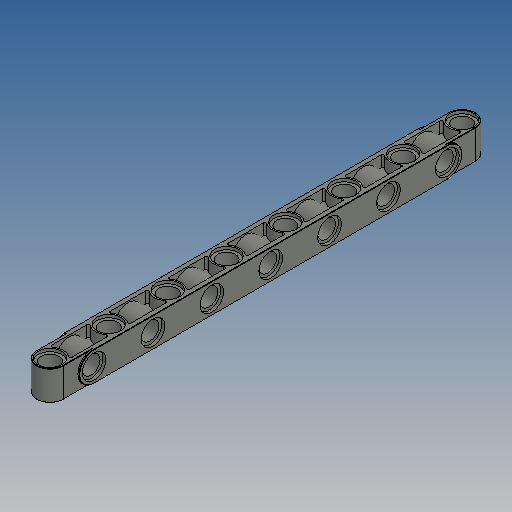
# Autodesk Inventor part: 6330585-Black
Saved by Autodesk Inventor 2025 (Build 290162010, 162A)
## iProperties
Created: 2012-03-21
Part Number: 6330585-Black
Document SubType Name: Modeling
Designer: h.muther
Density: 1.06 g/cm^3
Material: ABS Plastic
Mass: 2.72969 g
Surface Area: 46.8865 cm^2
Volume: 2.57518 cm^3
Appearance: DkBluishGray
Description: Technic, Liftarm 11
Author: h.muther
Autodesk Inventor part; units mm, degrees
ref_plane "YZ Plane" through (0, 0, 0) normal (1, 0, 0) x (0, 1, 0)
ref_plane "XZ Plane" through (0, 0, 0) normal (0, 1, 0) x (-1, 0, 0)
ref_plane "XY Plane" through (0, 0, 0) normal (0, 0, 1) x (1, 0, 0)
sketch "Sketch1" plane through (0, 0, 0) normal (0, 0, 1) x (1, 0, 0)
  line L0 (3.6, -56) -> (3.6, 56)
  line L1 (-3.6, 56) -> (-3.6, -56)
  arc A0 (3.6, 56) -> (-3.6, 56) centre (0, 56) ccw
  arc A1 (-3.6, -56) -> (3.6, -56) centre (0, -56) ccw
  circle A2 centre (0, 56) radius 3.2
  circle A3 centre (0, 56) radius 2.4
  line L2 (2.8, 53.7373) -> (2.8, 42.2627)
  line L3 (-2.8, 53.7373) -> (-2.8, 42.2627)
  arc A4 (-2.8, 53.7373) -> (2.8, 53.7373) centre (0, 56) ccw
  arc A5 (2.8, 42.2627) -> (-2.8, 42.2627) centre (0, 40) ccw
  circle A6 centre (0, 40) radius 3.2
  circle A7 centre (0, 40) radius 2.4
  line L4 (2.8, 37.7373) -> (2.8, 26.2627)
  line L5 (-2.8, 37.7373) -> (-2.8, 26.2627)
  arc A8 (-2.8, 37.7373) -> (2.8, 37.7373) centre (0, 40) ccw
  arc A9 (2.8, 26.2627) -> (-2.8, 26.2627) centre (0, 24) ccw
  circle A10 centre (0, 24) radius 3.2
  circle A11 centre (0, 24) radius 2.4
  line L6 (2.8, 21.7373) -> (2.8, 10.2627)
  line L7 (-2.8, 21.7373) -> (-2.8, 10.2627)
  arc A12 (-2.8, 21.7373) -> (2.8, 21.7373) centre (0, 24) ccw
  arc A13 (2.8, 10.2627) -> (-2.8, 10.2627) centre (0, 8) ccw
  circle A14 centre (0, 8) radius 3.2
  circle A15 centre (0, 8) radius 2.4
  line L8 (2.8, 5.7373) -> (2.8, -5.7373)
  line L9 (-2.8, 5.7373) -> (-2.8, -5.7373)
  arc A16 (-2.8, 5.7373) -> (2.8, 5.7373) centre (0, 8) ccw
  arc A17 (2.8, -5.7373) -> (-2.8, -5.7373) centre (0, -8) ccw
  circle A18 centre (0, -8) radius 3.2
  circle A19 centre (0, -8) radius 2.4
  line L10 (2.8, -10.2627) -> (2.8, -21.7373)
  line L11 (-2.8, -10.2627) -> (-2.8, -21.7373)
  arc A20 (-2.8, -10.2627) -> (2.8, -10.2627) centre (0, -8) ccw
  arc A21 (2.8, -21.7373) -> (-2.8, -21.7373) centre (0, -24) ccw
  circle A22 centre (0, -24) radius 3.2
  circle A23 centre (0, -24) radius 2.4
  circle A24 centre (0, -40) radius 2.4
  circle A25 centre (0, -40) radius 3.2
  line L12 (2.8, -26.2627) -> (2.8, -37.7373)
  arc A26 (2.8, -37.7373) -> (-2.8, -37.7373) centre (0, -40) ccw
  arc A27 (-2.8, -26.2627) -> (2.8, -26.2627) centre (0, -24) ccw
  line L13 (-2.8, -26.2627) -> (-2.8, -37.7373)
  circle A28 centre (0, -56) radius 2.4
  circle A29 centre (0, -56) radius 3.2
  line L14 (2.8, -42.2627) -> (2.8, -53.7373)
  arc A30 (2.8, -53.7373) -> (-2.8, -53.7373) centre (0, -56) ccw
  arc A31 (-2.8, -42.2627) -> (2.8, -42.2627) centre (0, -40) ccw
  line L15 (-2.8, -42.2627) -> (-2.8, -53.7373)
  point P0 (0, 0)
  point P1 (-3.6, 0)
  dimension "d32" = 7.2
  dimension "d48" = 112
  dimension "d49" = 6.4
  dimension "d50" = 4.8
  dimension "d51" = 16
  dimension "d52" = 0.8
  dimension "d55" = 16
  constraints: 32 centre point, 32 end point, 32 point on circle, 17 coincident, 4 equal radius, 4 tangent, 3 horizontal alignment, 3 vertical, 2 vertical alignment, 1 midpoint, 1 parallel, 84 other
  measures "d32" diameter of A0
  measures "d48" distance of A1.centre A0.centre
  measures "d49" diameter of A2
  measures "d50" diameter of A3
  measures "d51" distance of A0.centre A5.centre
  measures "d52" distance between parallel lines of L1 L3
  measures "d55" distance of A7.centre A11.centre
extrude "Extrusion1" add sketch "Sketch1" along normal mid plane 8 contours A1 L1 A0 L0 | A2 | L2 A5 L3 A4 | A6 | L4 A9 L5 A8 | A10 | L6 A13 L7 A12 | A14 | L8 A17 L9 A16 | A18 | L10 A21 L11 A20 | A22 | A25 | L12 A26 L13 A27 | A29 | L14 A30 L15 A31
sketch "Sketch6" plane through (0, 0, 4) normal (0, 0, 1) x (1, 0, 0)
  line L0 (2.8, -10.2627) -> (2.8, -21.7373) projected
  arc A0 (-2.8, -10.2627) -> (2.8, -10.2627) centre (0, -8) ccw projected
  line L1 (-2.8, -10.2627) -> (-2.8, -21.7373) projected
  circle A1 centre (0, -24) radius 3.2 projected
  arc A2 (2.8, -21.7373) -> (-2.8, -21.7373) centre (0, -24) ccw projected
  circle A3 centre (0, -8) radius 3.2 projected
  arc A4 (2.8, -5.7373) -> (-2.8, -5.7373) centre (0, -8) ccw projected
  line L2 (-2.8, 5.7373) -> (-2.8, -5.7373) projected
  line L3 (2.8, 5.7373) -> (2.8, -5.7373) projected
  circle A5 centre (0, 8) radius 3.2 projected
  arc A6 (-2.8, 5.7373) -> (2.8, 5.7373) centre (0, 8) ccw projected
  arc A7 (2.8, 10.2627) -> (-2.8, 10.2627) centre (0, 8) ccw projected
  line L4 (-2.8, 21.7373) -> (-2.8, 10.2627) projected
  line L5 (2.8, 21.7373) -> (2.8, 10.2627) projected
  circle A8 centre (0, 24) radius 3.2 projected
  arc A9 (-2.8, 21.7373) -> (2.8, 21.7373) centre (0, 24) ccw projected
  line L6 (-2.8, 37.7373) -> (-2.8, 26.2627) projected
  arc A10 (2.8, 26.2627) -> (-2.8, 26.2627) centre (0, 24) ccw projected
  line L7 (2.8, 37.7373) -> (2.8, 26.2627) projected
  circle A11 centre (0, 40) radius 3.2 projected
  arc A12 (-2.8, 37.7373) -> (2.8, 37.7373) centre (0, 40) ccw projected
  arc A13 (2.8, 42.2627) -> (-2.8, 42.2627) centre (0, 40) ccw projected
  line L8 (-2.8, 53.7373) -> (-2.8, 42.2627) projected
  line L9 (2.8, 53.7373) -> (2.8, 42.2627) projected
  arc A14 (-2.8, 53.7373) -> (2.8, 53.7373) centre (0, 56) ccw projected
  circle A15 centre (0, 56) radius 3.2 projected
  circle A16 centre (0, -56) radius 2.4 projected
  circle A17 centre (0, -56) radius 3.2 projected
  line L10 (-2.8, -42.2627) -> (-2.8, -53.7373) projected
  arc A18 (2.8, -53.7373) -> (-2.8, -53.7373) centre (0, -56) ccw projected
  line L11 (2.8, -42.2627) -> (2.8, -53.7373) projected
  arc A19 (-2.8, -42.2627) -> (2.8, -42.2627) centre (0, -40) ccw projected
  circle A20 centre (0, -40) radius 3.2 projected
  arc A21 (2.8, -37.7373) -> (-2.8, -37.7373) centre (0, -40) ccw projected
  line L12 (2.8, -26.2627) -> (2.8, -37.7373) projected
  arc A22 (-2.8, -26.2627) -> (2.8, -26.2627) centre (0, -24) ccw projected
  line L13 (-2.8, -26.2627) -> (-2.8, -37.7373) projected
  circle A23 centre (0, -40) radius 2.4 projected
extrude "Extrusion7" cut sketch "Sketch6" against normal blind 0.8 contours A1 | A3 | A5 | A8 | A11 | A15 | A16 | A17 | A20 | A23
extrude "Extrusion8" cut sketch "Sketch6" against normal blind 3.1 contours L0 A2 L1 A0 | A4 L2 A6 L3 | A7 L4 A9 L5 | A12 L7 A10 L6 | A13 L8 A14 L9 | A19 L11 A18 L10 | A21 L13 A22 L12
mirror "Mirror1" about plane through (0, 0, 0) normal (0, 0, 1) of "Extrusion7", "Extrusion8"
fillet "Fillet2" radius 0.4 28 edges at (2.8, -10.2627, -2.45) (-2.8, -10.2627, -2.45) (-2.8, 5.7373, -2.45) (2.8, 5.7373, -2.45) (2.8, -5.7373, -2.45) (-2.8, -5.7373, -2.45) (-2.8, -21.7373, -2.45) (2.8, -21.7373, -2.45) (2.8, 10.2627, -2.45) (2.8, 21.7373, -2.45) (2.8, 26.2627, -2.45) (2.8, 37.7373, -2.45) (2.8, 42.2627, -2.45) (2.8, 53.7373, -2.45) (-2.8, 53.7373, -2.45) (-2.8, 42.2627, -2.45) (-2.8, 37.7373, -2.45) (-2.8, 26.2627, -2.45) (-2.8, 21.7373, -2.45) (-2.8, 10.2627, -2.45) (2.8, -26.2627, -2.45) (2.8, -42.2627, -2.45) (-2.8, -42.2627, -2.45) (-2.8, -26.2627, -2.45) (-2.8, -37.7373, -2.45) (2.8, -37.7373, -2.45) (2.8, -53.7373, -2.45) (-2.8, -53.7373, -2.45)
fillet "Fillet2" radius 0.1 4 edges at (0, 59.6, -4) (-3.6, 0, -4) (0, -59.6, -4) (3.6, 0, -4)
mirror "Spiegeln2" about plane through (0, 0, 0) normal (0, 0, 1) of "Fillet2"
sketch "Skizze9" plane through (-3.6, -56, -3.9) normal (-1, 0, 0) x (0, 0, 1)
  line L0 (3.9, 104) -> (3.9, 8) construction
  line L1 (-0.1, 104) -> (-0.1, 8)
  line L2 (7.9, 8) -> (7.9, 104)
  arc A0 (7.9, 104) -> (-0.1, 104) centre (3.9, 104) ccw
  arc A1 (-0.1, 8) -> (7.9, 8) centre (3.9, 8) ccw
  line L3 (7.9, 0) -> (7.9, 112) projected
  line L4 (7.9, 35.2) -> (7.9, 44.8) projected
  line L5 (4.8, 12.8) -> (4.8, 3.2) projected
  point P0 (3.9, 56)
  point P1 (7.9, 40)
  point P2 (4.8, 8)
  constraints: 8 end point, 4 point on circle, 4 tangent, 3 midpoint, 2 centre point, 1 collinear, 1 horizontal alignment, 1 parallel
extrude "Extrusion9" add sketch "Skizze9" along normal blind 0.4
delete faces "Fläche löschen1" heal yes whole lump no faces at (-3.6, -16, 3.9333) (-3.6, -16, -3.9333)
fillet "Rundung3" radius 0.1 4 edges at (-4, 52, 0) (-4, 0, -4) (-4, -52, 0) (-4, 0, 4)
mirror "Spiegeln3" about plane through (0, 0, 0) normal (1, 0, 0) of "Extrusion9", "Fläche löschen1", "Rundung3"
sketch "Skizze10" plane through (-4, -56, -3.9) normal (-1, 0, 0) x (0, 0, 1)
  circle A0 centre (3.9, 8) radius 3.6
  arc A1 (0, 8) -> (7.8, 8) centre (3.9, 8) ccw projected
  dimension "d66" = 7.2
  constraints: 1 centre point, 1 coincident, 1 concentric
  measures "d66" diameter of A0
extrude "Extrusion10" add sketch "Skizze10" against normal up to surface (8 mm away)
sketch "Skizze11" plane through (-4, -56, -3.9) normal (-1, 0, 0) x (0, 0, 1)
  circle A0 centre (3.9, 8) radius 3.2
  arc A1 (0, 8) -> (7.8, 8) centre (3.9, 8) ccw projected
  point P0 (3.9, 56)
  dimension "d69" = 6.4
  constraints: 1 centre point, 1 concentric
  measures "d69" diameter of A0
extrude "Extrusion11" cut sketch "Skizze11" against normal blind 0.8
sketch "Skizze12" plane through (4, -48, 3.9) normal (1, 0, 0) x (0, 0, -1)
  circle A0 centre (3.9, 0) radius 3.2 projected
  point P0 (3.9, 48)
extrude "Extrusion12" cut sketch "Skizze12" against normal blind 0.8
sketch "Skizze13" plane through (3.2, -48, 0) normal (1, 0, 0) x (0, 0, -1)
  circle A0 centre (0, 0) radius 3.2 projected
  point P0 (0, 48)
  constraints: 1 coincident
hole "Bohrung1" at (3.2, -48, 0) direction (-1, 0, 0) diameter 4.8 end through all
pattern_linear "Rechteckige Anordnung1" count 7 spacing 16 along (0, 1, 0) of "Bohrung1", "Extrusion12", "Extrusion11", "Extrusion10"
body "Solid1"
